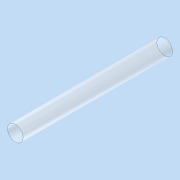
# Autodesk Inventor part: Cartridge-Plastic
Saved by Autodesk Inventor 2012 (Build 160160000, 160)
## iProperties
Created: 2014-10-01
Part Number: Cartridge-Plastic
Material: Default
Document SubType Name: Modeling
Designer: Jason
Density: 1 g/cm^3
Author: Jason
Autodesk Inventor part; units mm, degrees
ref_plane "YZ Plane" through (0, 0, 0) normal (1, 0, 0) x (0, 1, 0)
ref_plane "XZ Plane" through (0, 0, 0) normal (0, 1, 0) x (-1, 0, 0)
ref_plane "XY Plane" through (0, 0, 0) normal (0, 0, 1) x (1, 0, 0)
sketch "Sketch1" plane through (0, 0, 0) normal (0, 0, 1) x (1, 0, 0)
  circle A0 centre (0, 0) radius 4
  circle A1 centre (0, 0) radius 3.99
  dimension "d0" = 8
  dimension "d1" = 0.01
  constraints: 2 centre point, 2 coincident
  measures "d0" diameter of A0
  measures "d1" radial gap between concentric circles of A0 A1
extrude "Extrusion1" add sketch "Sketch1" along normal mid plane 76.66
body "Solid1"
